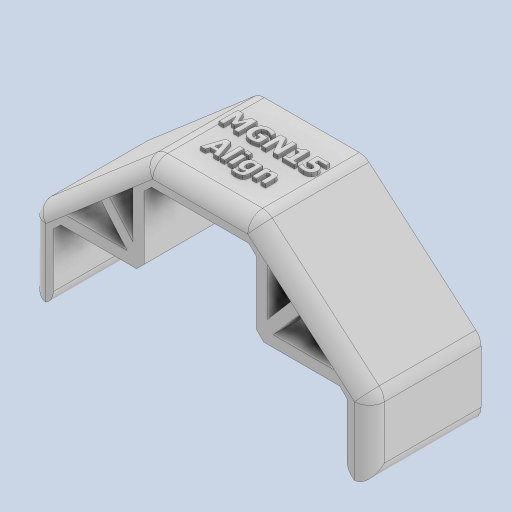
# Autodesk Inventor part: MGN15-AssemblyGuide
Saved by Autodesk Inventor 2023.2 (Build 272271000, 271)
## iProperties
Created: 2024-03-20
Part Number: MGN15-AssemblyGuide
Material: Generisch
Document SubType Name: Modeling
Designer: Nils Bade
Density: 1 g/cm^3
Appearance: Vorgabe
Author: Nils Bade
Autodesk Inventor part; units mm, degrees
ref_plane "YZ Plane" through (0, 0, 0) normal (1, 0, 0) x (0, 1, 0)
ref_plane "XZ Plane" through (0, 0, 0) normal (0, 1, 0) x (-1, 0, 0)
ref_plane "XY Plane" through (0, 0, 0) normal (0, 0, 1) x (1, 0, 0)
sketch "Skizze1" plane through (0, 0, 0) normal (0, 0, 1) x (1, 0, 0)
  line L0 (-19.75, 20) -> (19.75, 20) construction
  line L1 (19.75, 20) -> (19.75, -20) construction
  line L2 (19.75, -20) -> (-19.75, -20) construction
  line L3 (-19.75, -20) -> (-19.75, 20) construction
  line L4 (-19.75, 20) -> (19.75, -20) construction
  line L5 (19.75, 20) -> (-19.75, -20) construction
  line L6 (-7.55, 20) -> (7.55, 20) construction
  line L7 (7.55, 20) -> (7.55, 30.5) construction
  line L8 (7.55, 30.5) -> (-7.55, 30.5) construction
  line L9 (-7.55, 30.5) -> (-7.55, 20) construction
  line L10 (0, 30.5) -> (-7.55, 30.5)
  line L11 (-7.55, 30.5) -> (-7.55, 20)
  line L12 (-7.55, 20) -> (-19.75, 20)
  line L13 (-19.75, 20) -> (-19.75, 10)
  line L14 (-22.75, 10) -> (-19.75, 10)
  line L15 (-22.75, 10) -> (-22.75, 20.0568)
  line L16 (-22.75, 20.0568) -> (-7.1302, 33.5)
  line L17 (-7.1302, 33.5) -> (0, 33.5)
  line L18 (0, 33.5) -> (0, 30.5)
  line L19 (-7.55, 30.5) -> (-19.75, 20)
  line L20 (-8.5395, 20) -> (-13.3099, 25.5427)
  line L21 (-12.173, 26.5212) -> (-7.55, 21.1497)
  line L22 (-7.55, 20) -> (-12.7414, 26.032) construction
  line L23 (-9.8305, 21.5) -> (-18.0071, 21.5)
  line L24 (-9.05, 22.8926) -> (-9.05, 29.209)
  point P0 (0, 0)
  point P1 (0, 20)
  point P2 (-13.9561, 25.2884)
  dimension "d0" = 39.5
  dimension "d1" = 40
  dimension "d2" = 15.1
  dimension "d3" = 10.5
  dimension "d4" = 3
  dimension "d5" = 10
  dimension "d6" = 3
  dimension "d8" = 2
  dimension "d9" = 1.5
  dimension "d10" = 1.5
  dimension "d11" = 1.5
  constraints: 50 end point, 11 point on line, 8 perpendicular, 7 parallel, 5 midpoint, 2 collinear, 2 horizontal, 1 vertical, 1 other
  measures "d0" distance of L1.end L2.end
  measures "d1" distance of L0.end L1.end
  measures "d2" distance of L8.end L7.end
  measures "d3" distance of L7.end L6.end
  measures "d4" distance between parallel lines of L15 L13
  measures "d5" distance between parallel lines of L12 L14
  measures "d6" distance between parallel lines of L8 L17
  measures "d8" distance between parallel lines of L16 L19
  measures "d9" distance between parallel lines of L20 L21
  measures "d10" distance between parallel lines of L24 L9
  measures "d11" distance between parallel lines of L0 L23
extrude "Extrusion1" add sketch "Skizze1" along normal blind 15 contours L10 L19 L13 L14 L15 L16 L17 L18 | L11 L21 L24 L19 | L11 L12 L20 L19 L21 | L12 L19 L23 L20
chamfer "Fase3" distance 1 angle 45 3 edges at (-19.75, 20, 7.5) (-7.55, 30.5, 7.5) (-7.55, 20, 7.5)
fillet "Rundung2" radius 2 7 edges at (-22.75, 20.0568, 7.5) (-22.75, 15.0284, 15) (-22.75, 10, 7.5) (-7.1302, 33.5, 7.5) (-3.5651, 33.5, 15) (-19.75, 10, 7.5) (-14.9401, 26.7784, 15)
mirror "Spiegeln1" about plane through (0, 0, 0) normal (1, 0, 0)
sketch "Skizze2" plane through (-7.1302, 33.5, 15) normal (0, 1, 0) x (1, 0, 0)
  line L0 (0.7396, 15) -> (13.4791, 15) construction
  line L1 (13.4791, 15) -> (13.4791, 0.1101) construction
  line L2 (13.4791, 0.1101) -> (0.7396, 0.1101) construction
  line L3 (0.7396, 0.1101) -> (0.7396, 15) construction
  line L4 (3.534, 8.7116) -> (2.9, 8.7116)
  line L5 (2.9, 8.7116) -> (2.9, 10.3953)
  line L6 (2.9, 10.3953) -> (2.439, 9.3085)
  line L7 (2.439, 9.3085) -> (2.0026, 9.3085)
  line L8 (2.0026, 9.3085) -> (1.5415, 10.3953)
  line L9 (1.5415, 10.3953) -> (1.5415, 8.7116)
  line L10 (1.5415, 8.7116) -> (0.9405, 8.7116)
  line L11 (0.9405, 8.7116) -> (0.9405, 11.2516)
  line L12 (0.9405, 11.2516) -> (1.6753, 11.2516)
  line L13 (1.6753, 11.2516) -> (2.2393, 9.998)
  line L14 (2.2393, 9.998) -> (2.7992, 11.2516)
  line L15 (2.7992, 11.2516) -> (3.534, 11.2516)
  line L16 (3.534, 11.2516) -> (3.534, 8.7116)
  spline S0 degree 2 poles (6.181, 8.8557) (6.0143, 8.7877) (5.4812, 8.6581) (5.2218, 8.6581) knots 0 0 0 1 2 2 2
  spline S1 degree 2 poles (5.2218, 8.6581) (4.6229, 8.6581) (3.9127, 9.3497) (3.9127, 9.9836) knots 0 0 0 1 2 2 2
  spline S2 degree 2 poles (3.9127, 9.9836) (3.9127, 10.5806) (4.6229, 11.301) (5.2404, 11.301) knots 0 0 0 1 2 2 2
  spline S3 degree 2 poles (5.2404, 11.301) (5.5594, 11.301) (5.9587, 11.1795) (6.1707, 11.0766) knots 0 0 0 1 2 2 2
  line L17 (6.1707, 11.0766) -> (6.1707, 10.4797)
  line L18 (6.1707, 10.4797) -> (6.1131, 10.4797)
  spline S4 degree 2 poles (6.1131, 10.4797) (6.0678, 10.5147) (5.8949, 10.6485) (5.8126, 10.6938) knots 0 0 0 1 2 2 2
  spline S5 degree 2 poles (5.8126, 10.6938) (5.7179, 10.7493) (5.4668, 10.8276) (5.3268, 10.8276) knots 0 0 0 1 2 2 2
  spline S6 degree 2 poles (5.3268, 10.8276) (5.1642, 10.8276) (4.8946, 10.7246) (4.7896, 10.6197) knots 0 0 0 1 2 2 2
  spline S7 degree 2 poles (4.7896, 10.6197) (4.6887, 10.5167) (4.5714, 10.2018) (4.5714, 9.9939) knots 0 0 0 1 2 2 2
  spline S8 degree 2 poles (4.5714, 9.9939) (4.5714, 9.5493) (5.0181, 9.1253) (5.403, 9.1253) knots 0 0 0 1 2 2 2
  spline S9 degree 2 poles (5.403, 9.1253) (5.438, 9.1253) (5.5285, 9.1294) (5.5635, 9.1315) knots 0 0 0 1 2 2 2
  line L19 (5.5635, 9.1315) -> (5.5635, 9.6317)
  line L20 (5.5635, 9.6317) -> (5.0716, 9.6317)
  line L21 (5.0716, 9.6317) -> (5.0716, 10.1071)
  line L22 (5.0716, 10.1071) -> (6.181, 10.1071)
  line L23 (6.181, 10.1071) -> (6.181, 8.8557)
  line L24 (8.8384, 8.7116) -> (8.225, 8.7116)
  line L25 (8.225, 8.7116) -> (7.2452, 10.4818)
  line L26 (7.2452, 10.4818) -> (7.2452, 8.7116)
  line L27 (7.2452, 8.7116) -> (6.6627, 8.7116)
  line L28 (6.6627, 8.7116) -> (6.6627, 11.2516)
  line L29 (6.6627, 11.2516) -> (7.4449, 11.2516)
  line L30 (7.4449, 11.2516) -> (8.2558, 9.7963)
  line L31 (8.2558, 9.7963) -> (8.2558, 11.2516)
  line L32 (8.2558, 11.2516) -> (8.8384, 11.2516)
  line L33 (8.8384, 11.2516) -> (8.8384, 8.7116)
  line L34 (11.1025, 8.7116) -> (9.425, 8.7116)
  line L35 (9.425, 8.7116) -> (9.425, 9.1541)
  line L36 (9.425, 9.1541) -> (9.9602, 9.1541)
  line L37 (9.9602, 9.1541) -> (9.9602, 10.4982)
  line L38 (9.9602, 10.4982) -> (9.425, 10.4982)
  line L39 (9.425, 10.4982) -> (9.425, 10.9119)
  spline S10 degree 2 poles (9.425, 10.9119) (9.5423, 10.9119) (9.7749, 10.9428) (9.8449, 10.9758) knots 0 0 0 1 2 2 2
  spline S11 degree 2 poles (9.8449, 10.9758) (9.9252, 11.0169) (10.0157, 11.1548) (10.024, 11.2577) knots 0 0 0 1 2 2 2
  line L40 (10.024, 11.2577) -> (10.5797, 11.2577)
  line L41 (10.5797, 11.2577) -> (10.5797, 9.1541)
  line L42 (10.5797, 9.1541) -> (11.1025, 9.1541)
  line L43 (11.1025, 9.1541) -> (11.1025, 8.7116)
  spline S12 degree 2 poles (13.3832, 9.572) (13.3832, 9.3723) (13.2473, 9.0347) (13.1135, 8.9133) knots 0 0 0 1 2 2 2
  spline S13 degree 2 poles (13.1135, 8.9133) (12.9797, 8.7918) (12.6134, 8.6581) (12.3458, 8.6581) knots 0 0 0 1 2 2 2
  spline S14 degree 2 poles (12.3458, 8.6581) (12.0617, 8.6601) (11.6542, 8.7527) (11.5204, 8.8124) knots 0 0 0 1 2 2 2
  line L44 (11.5204, 8.8124) -> (11.5204, 9.3661)
  line L45 (11.5204, 9.3661) -> (11.578, 9.3661)
  spline S15 degree 2 poles (11.578, 9.3661) (11.6274, 9.3394) (11.7468, 9.2694) (11.8435, 9.2323) knots 0 0 0 1 2 2 2
  spline S16 degree 2 poles (11.8435, 9.2323) (11.9341, 9.1973) (12.1214, 9.15) (12.2346, 9.15) knots 0 0 0 1 2 2 2
  spline S17 degree 2 poles (12.2346, 9.15) (12.3334, 9.15) (12.564, 9.1994) (12.6339, 9.2653) knots 0 0 0 1 2 2 2
  spline S18 degree 2 poles (12.6339, 9.2653) (12.6854, 9.3167) (12.743, 9.4423) (12.743, 9.5473) knots 0 0 0 1 2 2 2
  spline S19 degree 2 poles (12.743, 9.5473) (12.743, 9.6378) (12.6689, 9.7654) (12.6092, 9.8046) knots 0 0 0 1 2 2 2
  spline S20 degree 2 poles (12.6092, 9.8046) (12.5228, 9.8622) (12.2758, 9.8951) (12.1873, 9.8951) knots 0 0 0 1 2 2 2
  spline S21 degree 2 poles (12.1873, 9.8951) (12.0473, 9.8951) (11.7818, 9.8498) (11.685, 9.8251) knots 0 0 0 1 2 2 2
  line L46 (11.685, 9.8251) -> (11.6295, 9.8251)
  line L47 (11.6295, 9.8251) -> (11.6295, 11.2516)
  line L48 (11.6295, 11.2516) -> (13.3132, 11.2516)
  line L49 (13.3132, 11.2516) -> (13.3132, 10.772)
  line L50 (13.3132, 10.772) -> (12.2326, 10.772)
  line L51 (12.2326, 10.772) -> (12.2326, 10.35)
  spline S22 degree 2 poles (12.2326, 10.35) (12.284, 10.3541) (12.4261, 10.3583) (12.4652, 10.3583) knots 0 0 0 1 2 2 2
  spline S23 degree 2 poles (12.4652, 10.3583) (12.6484, 10.3583) (12.9571, 10.2842) (13.0786, 10.208) knots 0 0 0 1 2 2 2
  spline S24 degree 2 poles (13.0786, 10.208) (13.2226, 10.1133) (13.3832, 9.7984) (13.3832, 9.572) knots 0 0 0 1 2 2 2
  line L52 (2.6324, 4.5295) -> (3.4908, 7.0695)
  line L53 (3.4908, 7.0695) -> (4.1865, 7.0695)
  line L54 (4.1865, 7.0695) -> (5.0448, 4.5295)
  line L55 (5.0448, 4.5295) -> (4.3882, 4.5295)
  line L56 (4.3882, 4.5295) -> (4.2297, 5.0482)
  line L57 (4.2297, 5.0482) -> (3.4311, 5.0482)
  line L58 (3.4311, 5.0482) -> (3.2705, 4.5295)
  line L59 (3.2705, 4.5295) -> (2.6324, 4.5295)
  line L60 (4.0897, 5.5093) -> (3.8304, 6.3491)
  line L61 (3.8304, 6.3491) -> (3.569, 5.5093)
  line L62 (3.569, 5.5093) -> (4.0897, 5.5093)
  line L63 (5.8599, 4.5295) -> (5.263, 4.5295)
  line L64 (5.263, 4.5295) -> (5.263, 7.1827)
  line L65 (5.263, 7.1827) -> (5.8599, 7.1827)
  line L66 (5.8599, 7.1827) -> (5.8599, 4.5295)
  line L67 (6.9138, 4.5295) -> (6.3169, 4.5295)
  line L68 (6.3169, 4.5295) -> (6.3169, 6.4459)
  line L69 (6.3169, 6.4459) -> (6.9138, 6.4459)
  line L70 (6.9138, 6.4459) -> (6.9138, 4.5295)
  line L71 (6.9323, 6.7196) -> (6.3004, 6.7196)
  line L72 (6.3004, 6.7196) -> (6.3004, 7.1848)
  line L73 (6.3004, 7.1848) -> (6.9323, 7.1848)
  line L74 (6.9323, 7.1848) -> (6.9323, 6.7196)
  spline S25 degree 2 poles (9.1121, 4.7498) (9.1121, 4.4842) (8.9577, 4.1117) (8.826, 4.0088) knots 0 0 0 1 2 2 2
  spline S26 degree 2 poles (8.826, 4.0088) (8.6922, 3.9038) (8.3217, 3.8091) (8.0953, 3.8091) knots 0 0 0 1 2 2 2
  spline S27 degree 2 poles (8.0953, 3.8091) (7.9039, 3.8091) (7.5601, 3.8585) (7.4346, 3.8914) knots 0 0 0 1 2 2 2
  line L75 (7.4346, 3.8914) -> (7.4346, 4.371)
  line L76 (7.4346, 4.371) -> (7.5045, 4.371)
  spline S28 degree 2 poles (7.5045, 4.371) (7.5478, 4.3546) (7.6692, 4.3134) (7.731, 4.2969) knots 0 0 0 1 2 2 2
  spline S29 degree 2 poles (7.731, 4.2969) (7.8051, 4.2784) (7.945, 4.2537) (8.0171, 4.2537) knots 0 0 0 1 2 2 2
  spline S30 degree 2 poles (8.0171, 4.2537) (8.1694, 4.2537) (8.3711, 4.3155) (8.4226, 4.3731) knots 0 0 0 1 2 2 2
  spline S31 degree 2 poles (8.4226, 4.3731) (8.474, 4.4328) (8.5152, 4.5933) (8.5152, 4.7168) knots 0 0 0 1 2 2 2
  line L77 (8.5152, 4.7168) -> (8.5152, 4.7518)
  spline S32 degree 2 poles (8.5152, 4.7518) (8.4143, 4.6633) (8.1509, 4.5563) (8.0109, 4.5563) knots 0 0 0 1 2 2 2
  spline S33 degree 2 poles (8.0109, 4.5563) (7.6383, 4.5563) (7.2349, 5.04) (7.2349, 5.5361) knots 0 0 0 1 2 2 2
  spline S34 degree 2 poles (7.2349, 5.5361) (7.2349, 5.7604) (7.3584, 6.1186) (7.4696, 6.2441) knots 0 0 0 1 2 2 2
  spline S35 degree 2 poles (7.4696, 6.2441) (7.5766, 6.3656) (7.875, 6.4973) (8.0377, 6.4973) knots 0 0 0 1 2 2 2
  spline S36 degree 2 poles (8.0377, 6.4973) (8.1838, 6.4973) (8.4164, 6.4232) (8.5111, 6.3615) knots 0 0 0 1 2 2 2
  line L78 (8.5111, 6.3615) -> (8.5337, 6.4459)
  line L79 (8.5337, 6.4459) -> (9.1121, 6.4459)
  line L80 (9.1121, 6.4459) -> (9.1121, 4.7498)
  line L81 (8.5152, 5.1326) -> (8.5152, 6.0012)
  spline S37 degree 2 poles (8.5152, 6.0012) (8.472, 6.0218) (8.3423, 6.0486) (8.2764, 6.0486) knots 0 0 0 1 2 2 2
  spline S38 degree 2 poles (8.2764, 6.0486) (8.0624, 6.0486) (7.8462, 5.7707) (7.8462, 5.5217) knots 0 0 0 1 2 2 2
  spline S39 degree 2 poles (7.8462, 5.5217) (7.8462, 5.3982) (7.8792, 5.2253) (7.9224, 5.1594) knots 0 0 0 1 2 2 2
  spline S40 degree 2 poles (7.9224, 5.1594) (7.9656, 5.0935) (8.1035, 5.0276) (8.2106, 5.0276) knots 0 0 0 1 2 2 2
  spline S41 degree 2 poles (8.2106, 5.0276) (8.2908, 5.0276) (8.4452, 5.0832) (8.5152, 5.1326) knots 0 0 0 1 2 2 2
  line L82 (11.3619, 4.5295) -> (10.7609, 4.5295)
  line L83 (10.7609, 4.5295) -> (10.7609, 5.4784)
  spline S42 degree 2 poles (10.7609, 5.4784) (10.7609, 5.5958) (10.7423, 5.8263) (10.7176, 5.8798) knots 0 0 0 1 2 2 2
  spline S43 degree 2 poles (10.7176, 5.8798) (10.6868, 5.9457) (10.5715, 6.0012) (10.4727, 6.0012) knots 0 0 0 1 2 2 2
  spline S44 degree 2 poles (10.4727, 6.0012) (10.4006, 6.0012) (10.2504, 5.9457) (10.166, 5.886) knots 0 0 0 1 2 2 2
  line L84 (10.166, 5.886) -> (10.166, 4.5295)
  line L85 (10.166, 4.5295) -> (9.5691, 4.5295)
  line L86 (9.5691, 4.5295) -> (9.5691, 6.4459)
  line L87 (9.5691, 6.4459) -> (10.166, 6.4459)
  line L88 (10.166, 6.4459) -> (10.166, 6.2338)
  spline S45 degree 2 poles (10.166, 6.2338) (10.3121, 6.3573) (10.59, 6.4973) (10.7588, 6.4973) knots 0 0 0 1 2 2 2
  spline S46 degree 2 poles (10.7588, 6.4973) (11.0511, 6.4973) (11.3619, 6.1268) (11.3619, 5.7769) knots 0 0 0 1 2 2 2
  line L89 (11.3619, 5.7769) -> (11.3619, 4.5295)
  point P0 (7.1302, 15)
  constraints: 2 other
extrude "Extrusion2" add sketch "Skizze2" along normal blind 0.5
